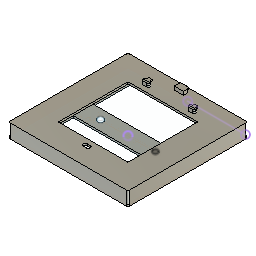
PanaThermoMount (Autodesk Fusion 360 design; units mm, degrees)
part number: 2025-10-30-14-12-04-186
Autodesk Fusion 360 part; units mm, degrees
sketch "MainBoardMount" plane through (0, 0, 0) normal (0, 0, 1) x (1, 0, 0)
  line L0 (0, 60) -> (-58, 60)
  line L1 (-60, 58) -> (-60, -58)
  line L2 (-58, -60) -> (0, -60)
  line L3 (0, 55.6) -> (0, 60)
  line L4 (0, -60) -> (0, -43.8)
  line L5 (0, -39.1) -> (0, 50.6)
  line L6 (0, 60) -> (58, 60)
  line L7 (60, 58) -> (60, -58)
  line L8 (0, -39.1) -> (0, 50.6)
  line L9 (58, -60) -> (0, -60)
  line L10 (0, 55.6) -> (0, 60)
  line L11 (0, -60) -> (0, -43.8)
  arc A0 (60, 58) -> (58, 60) centre (58, 58) ccw
  arc A1 (-58, 60) -> (-60, 58) centre (-58, 58) ccw
  arc A2 (-60, -58) -> (-58, -60) centre (-58, -58) ccw
  arc A3 (58, -60) -> (60, -58) centre (58, -58) ccw
  arc A4 (-24.65, 43.6) -> (-26.6, 41.65) centre (-24.65, 41.65) ccw
  arc A5 (-26.6, 41.65) -> (-24.65, 39.7) centre (-24.65, 41.65) ccw
  line L12 (-24.65, 39.7) -> (-21.35, 39.7)
  arc A6 (-21.35, 39.7) -> (-19.4, 41.65) centre (-21.35, 41.65) ccw
  arc A7 (-19.4, 41.65) -> (-21.35, 43.6) centre (-21.35, 41.65) ccw
  line L13 (-21.35, 43.6) -> (-24.65, 43.6)
  line L14 (21.35, 43.6) -> (24.65, 43.6)
  arc A8 (26.6, 41.65) -> (24.65, 43.6) centre (24.65, 41.65) ccw
  arc A9 (24.65, 39.7) -> (26.6, 41.65) centre (24.65, 41.65) ccw
  line L15 (24.65, 39.7) -> (21.35, 39.7)
  arc A10 (19.4, 41.65) -> (21.35, 39.7) centre (21.35, 41.65) ccw
  arc A11 (21.35, 43.6) -> (19.4, 41.65) centre (21.35, 41.65) ccw
  line L16 (0, 55.2) -> (4.6, 55.2)
  line L17 (4.6, 55.2) -> (4.6, 51)
  line L18 (4.6, 51) -> (0, 51)
  line L19 (-4.6, 51) -> (0, 51)
  line L20 (-4.6, 55.2) -> (-4.6, 51)
  line L21 (0, 55.2) -> (-4.6, 55.2)
  line L22 (0, -39.5) -> (1.65, -39.5)
  arc A12 (3.6, -41.45) -> (1.65, -39.5) centre (1.65, -41.45) ccw
  arc A13 (1.65, -43.4) -> (3.6, -41.45) centre (1.65, -41.45) ccw
  line L23 (1.65, -43.4) -> (0, -43.4)
  line L24 (-1.65, -43.4) -> (0, -43.4)
  arc A14 (-3.6, -41.45) -> (-1.65, -43.4) centre (-1.65, -41.45) ccw
  arc A15 (-1.65, -39.5) -> (-3.6, -41.45) centre (-1.65, -41.45) ccw
  line L25 (0, -39.5) -> (-1.65, -39.5)
  point P0 (-60, -60)
  point P1 (-19, 44)
  point P2 (-27, 44)
  point P3 (-27, 39.3)
  point P4 (-4, -39.1)
  point P5 (-4, -43.8)
  point P6 (27, 44)
  point P7 (4, -43.8)
  point P8 (27, 39.3)
  point P9 (4, -39.1)
  point P10 (19, 44)
  dimension "d21" = 120
  dimension "d24" = 4.7
  dimension "d25" = 8
  dimension "d26" = 60
  dimension "d28" = 4.7
  dimension "d29" = 4
  dimension "d35" = 2
  constraint perpendicular L0 L1
  constraint parallel L0 L2
  constraint parallel L1 L4
  constraint horizontal L0
  constraint coincident L3.start L4
  constraint coincident L5.start L4
  constraint collinear L3 L4
  constraint collinear L4 L5
  constraint symmetric L0.start L5 L3.end
  constraint symmetric L2.end L5 L4.start
  constraint symmetric P1 L5 P10
  constraint symmetric P2 L5 P6
  constraint symmetric P3 L5 P8
  constraint symmetric L3.start L5 L10.start
  constraint symmetric L8.end L5 L5.end
  constraint symmetric L8.start L5 L5.start
  constraint symmetric P4 L5 P9
  constraint symmetric P5 L5 P7
  constraint symmetric L4.end L5 L11.end
  constraint tangent L6 A0
  constraint tangent L7 A0
  constraint tangent L0 A1
  constraint tangent L1 A1
  constraint equal A0 A1
  constraint coincident P0 L1
  constraint coincident P0 L2
  constraint tangent L1 A2
  constraint tangent L2 A2
  constraint equal A0 A2
  constraint tangent L7 A3
  constraint tangent L9 A3
  constraint equal A0 A3
  constraint tangent L22 A12
  constraint tangent L24 A14
  constraint tangent A12 A13
  constraint tangent A13 L23
  constraint tangent A14 A15
  constraint tangent A15 L25
  constraint tangent A4 L13
  constraint tangent A4 A5
  constraint tangent A5 L12
  constraint tangent A6 A7
  constraint tangent L12 A6
  constraint tangent A7 L13
  constraint tangent L14 A11
  constraint tangent L14 A8
  constraint tangent L15 A10
  constraint tangent A8 A9
  constraint tangent A9 L15
  constraint tangent A10 A11
  measures "d21" distance of L0.start L2.end
  measures "d24" distance of P2 P3
  measures "d25" distance of P1 P2
  measures "d26" distance of P0 L2.end
  measures "d28" distance of P4 P5
  measures "d29" distance of L5.start P4
  measures "d35" radius of A0
extrude "Extrude5" add sketch "MainBoardMount" along normal blind 2
sketch "MountingPoints" plane through (0, 0, 2) normal (0, 0, 1) x (-1, 0, 0)
  arc A0 (-24.65, -39.7) -> (-24.65, -43.6) centre (-24.65, -41.65) ccw
  line L0 (-24.65, -39.7) -> (-21.35, -39.7)
  arc A1 (-21.35, -43.6) -> (-21.35, -39.7) centre (-21.35, -41.65) ccw
  line L1 (-21.35, -43.6) -> (-24.65, -43.6)
  line L2 (24.65, -43.6) -> (21.35, -43.6)
  arc A2 (21.35, -39.7) -> (21.35, -43.6) centre (21.35, -41.65) ccw
  line L3 (21.35, -39.7) -> (24.65, -39.7)
  arc A3 (24.65, -43.6) -> (24.65, -39.7) centre (24.65, -41.65) ccw
  arc A4 (-1.65, 43.4) -> (-1.65, 39.5) centre (-1.65, 41.45) ccw
  line L4 (-1.65, 43.4) -> (1.65, 43.4)
  arc A5 (1.65, 39.5) -> (1.65, 43.4) centre (1.65, 41.45) ccw
  line L5 (1.65, 39.5) -> (-1.65, 39.5)
  line L6 (4.6, -55.2) -> (-4.6, -55.2)
  line L7 (-4.6, -55.2) -> (-4.6, -51)
  line L8 (-4.6, -51) -> (4.6, -51)
  line L9 (4.6, -51) -> (4.6, -55.2)
  line L10 (-58, -60) -> (58, -60)
  arc A6 (58, -60) -> (60, -58) centre (58, -58) ccw
  line L11 (60, -58) -> (60, 58)
  arc A7 (60, 58) -> (58, 60) centre (58, 58) ccw
  line L12 (58, 60) -> (-58, 60)
  arc A8 (-58, 60) -> (-60, 58) centre (-58, 58) ccw
  line L13 (-60, 58) -> (-60, -58)
  arc A9 (-60, -58) -> (-58, -60) centre (-58, -58) ccw
extrude "Extrude6" add sketch "MountingPoints" along normal blind 3.5 and the other way blind 2 contours A0 L0 A1 L1 | L2 A2 L3 A3 | L6 L7 L8 L9
sketch "TopmostMountHolder" plane through (0, 55.2, 0) normal (0, 1, 0) x (-1, 0, 0)
  line L0 (-4.6, 2) -> (4.6, 2)
  line L1 (4.6, 2) -> (4.6, 5.5)
  line L2 (4.6, 5.5) -> (-4.6, 5.5)
  line L3 (-4.6, 5.5) -> (-4.6, 2)
  line L4 (-4.6, 5.5) -> (4.6, 5.5)
  line L5 (4.6, 5.5) -> (4.6, 3.75)
  line L6 (4.6, 3.75) -> (-4.6, 3.75)
  line L7 (-4.6, 3.75) -> (-4.6, 5.5)
  dimension "d53" = 1.75
  constraint horizontal L4
  constraint vertical L5
  constraint horizontal L6
  constraint vertical L7
  constraint midpoint L1 L5.end
  constraint coincident L2.end L3.start
  measures "d53" distance of L2.end L6.end
extrude "Extrude7" add sketch "TopmostMountHolder" along normal blind 2 contours L1 L2 L3 L4 L5 L6 L7
fillet "Fillet1" radius 1 1 edges at (0, 57.2, 3.75)
fillet "Fillet2" radius 1 6 edges at (-4.6, 55.7, 3.75) (-4.6, 56.9071, 4.0429) (-4.6, 57.2, 5.125) (4.6, 57.2, 5.125) (4.6, 56.9071, 4.0429) (4.6, 55.7, 3.75)
sketch "FilletedMountHolders" plane through (0, 43.6, 0) normal (0, 1, 0) x (-1, 0, 0)
  line L0 (-24.65, 2) -> (-21.35, 2)
  line L1 (-21.35, 2) -> (-21.35, 5.5)
  line L2 (-21.35, 5.5) -> (-24.65, 5.5)
  line L3 (-24.65, 5.5) -> (-24.65, 2)
ref_plane "WorkPlane1" through (-23, 41.65, 3.75) normal (0, 0, 1) x (-1, 0, 0)
split_face "SplitFace1" 2 faces at (-24.7472, 43.5976, 3.1667) (-19.6147, 40.7604, 3.1667) by plane through (-23, 41.65, 3.75) normal (0, 0, 1)
split_face "SplitFace2" 3 faces at (21.2528, 43.5976, 3.1667) (25.4074, 43.4469, 3.1667) (-22.45, 43.6, 2.5833) by plane through (-23, 41.65, 3.75) normal (0, 0, 1)
split_face "SplitFace3" 1 faces at (22.45, 43.6, 4.3333) by plane through (-23, 41.65, 3.75) normal (0, 0, 1)
ref_plane "WorkPlane2" through (23, 41.65, 3.75) normal (0, -1, 0) x (1, 0, 0)
split_face "SplitFace4" 3 faces at (22.45, 42.3, 5.5) (20.4174, 43.3625, 4.3333) (24.8442, 39.7097, 4.3333) by plane through (23, 41.65, 3.75) normal (0, -1, 0)
split_face "SplitFace5" 2 faces at (22.45, 43.6, 4.3333) (22.45, 43.6, 2.5833) by plane through (-23, 41.65, 3.75) normal (0, 0, 1)
split_face "SplitFace6" 3 faces at (-20.1726, 40.0956, 4.3333) (-23.55, 42.3, 5.5) (-26.0459, 43.0116, 4.3333) by plane through (23, 41.65, 3.75) normal (0, -1, 0)
move_face "OffsetFaces1" offset 2 1 faces at (22.45, 43.6, 4.3333)
move_face "OffsetFaces2" offset 2 1 faces at (-23.55, 43.6, 4.3333)
fillet "Fillet3" radius 1 2 edges at (-23, 45.6, 3.75) (23, 45.6, 3.75)
sketch "BackHole" plane through (0, 0, 0) normal (0, 0, -1) x (1, 0, 0)
  arc A0 (1.65, 39.5) -> (1.65, 43.4) centre (1.65, 41.45) ccw
  line L0 (1.65, 39.5) -> (-1.65, 39.5)
  arc A1 (-1.65, 43.4) -> (-1.65, 39.5) centre (-1.65, 41.45) ccw
  line L1 (-1.65, 43.4) -> (1.65, 43.4)
  line L2 (-58, -60) -> (58, -60)
  arc A2 (58, -60) -> (60, -58) centre (58, -58) ccw
  line L3 (60, -58) -> (60, 58)
  arc A3 (60, 58) -> (58, 60) centre (58, 58) ccw
  line L4 (58, 60) -> (-58, 60)
  arc A4 (-58, 60) -> (-60, 58) centre (-58, 58) ccw
  line L5 (-60, 58) -> (-60, -58)
  arc A5 (-60, -58) -> (-58, -60) centre (-58, -58) ccw
  line L6 (35, -35) -> (-35, -35)
  line L7 (-35, -35) -> (-35, 35)
  line L8 (-35, 35) -> (35, 35)
  line L9 (35, 35) -> (35, -35)
  constraint horizontal L6
  constraint vertical L7
  constraint horizontal L8
  constraint vertical L9
extrude "Extrude8" cut sketch "BackHole" against normal blind 2 contours L6 L7 L8 L9
sketch "Wall" plane through (0, 0, 0) normal (0, 0, -1) x (1, 0, 0)
  line L0 (-35, -35) -> (-35, 35)
  line L1 (-35, 35) -> (35, 35)
  line L2 (35, 35) -> (35, -35)
  line L3 (35, -35) -> (-35, -35)
  arc A0 (1.65, 39.5) -> (1.65, 43.4) centre (1.65, 41.45) ccw
  line L4 (1.65, 39.5) -> (-1.65, 39.5)
  arc A1 (-1.65, 43.4) -> (-1.65, 39.5) centre (-1.65, 41.45) ccw
  line L5 (-1.65, 43.4) -> (1.65, 43.4)
  line L6 (-58, -60) -> (58, -60)
  arc A2 (58, -60) -> (60, -58) centre (58, -58) ccw
  line L7 (60, -58) -> (60, 58)
  arc A3 (60, 58) -> (58, 60) centre (58, 58) ccw
  line L8 (58, 60) -> (-58, 60)
  arc A4 (-58, 60) -> (-60, 58) centre (-58, 58) ccw
  line L9 (-60, 58) -> (-60, -58)
  arc A5 (-60, -58) -> (-58, -60) centre (-58, -58) ccw
  line L10 (58, -58) -> (-58, -58)
  line L11 (-58, -58) -> (-58, 58)
  line L12 (-58, 58) -> (58, 58)
  line L13 (58, 58) -> (58, -58)
  dimension "d63" = 2
  dimension "d64" = 2
  constraint horizontal L10
  constraint vertical L11
  constraint horizontal L12
  constraint vertical L13
  constraint coincident A4.centre L11.end
  constraint coincident A2.centre L10.start
  measures "d63" distance of L6 L10
  measures "d64" distance of L7 L13
extrude "Extrude9" add sketch "Wall" along normal blind 10 contours L6 A2 L7 A3 L8 A4 L9 A5
sketch "BottomPlane" plane through (0, 0, -10) normal (0, 0, -1) x (1, 0, 0)
  line L0 (-58, 58) -> (58, 58)
  line L1 (58, 58) -> (58, -58)
  line L2 (58, -58) -> (-58, -58)
  line L3 (-58, -58) -> (-58, 58)
  arc A0 (-60, -58) -> (-58, -60) centre (-58, -58) ccw
  line L4 (-58, -60) -> (58, -60)
  arc A1 (58, -60) -> (60, -58) centre (58, -58) ccw
  line L5 (60, -58) -> (60, 58)
  arc A2 (60, 58) -> (58, 60) centre (58, 58) ccw
  line L6 (58, 60) -> (-58, 60)
  arc A3 (-58, 60) -> (-60, 58) centre (-58, 58) ccw
  line L7 (-60, 58) -> (-60, -58)
  line L8 (58, -60) -> (-58, -60)
  line L9 (-60, -58) -> (-60, 58)
  line L10 (-58, 60) -> (58, 60)
  line L11 (60, 58) -> (60, -58)
  arc A4 (-60, -58) -> (-58, -60) centre (-58, -58) ccw
  arc A5 (58, -60) -> (60, -58) centre (58, -58) ccw
  arc A6 (60, 58) -> (58, 60) centre (58, 58) ccw
  arc A7 (-58, 60) -> (-60, 58) centre (-58, 58) ccw
  point P0 (60, -60)
  point P1 (-60, -60)
  point P2 (60, 60)
  dimension "d67" = 120
  dimension "d68" = 120
  dimension "d69" = 2
  constraint horizontal L8
  constraint vertical L9
  constraint horizontal L10
  constraint vertical L11
  constraint coincident P1 L8
  constraint coincident P1 L9
  constraint tangent L8 A4
  constraint tangent L9 A4
  constraint coincident P0 L8
  constraint coincident P0 L11
  constraint tangent L8 A5
  constraint tangent L11 A5
  constraint equal A4 A5
  constraint coincident P2 L10
  constraint coincident P2 L11
  constraint tangent L10 A6
  constraint tangent L11 A6
  constraint equal A4 A6
  constraint tangent L9 A7
  constraint tangent L10 A7
  constraint equal A4 A7
  measures "d67" distance of P0 P1
  measures "d68" distance of P0 P2
  measures "d69" radius of A4
extrude "Extrude10" add sketch "BottomPlane" along normal blind 2 contours L0 L1 L2 L3 | A0 L4 A1 L5 A2 L6 A3 L7 L8 L9 L10 L11 A4 A5 A6 A7
sketch "MountingHoles" plane through (0, 0, -10) normal (0, 0, 1) x (-1, 0, 0)
  line L0 (58, -58) -> (58, 58)
  line L1 (58, 58) -> (-58, 58)
  line L2 (-58, 58) -> (-58, -58)
  line L3 (-58, -58) -> (58, -58)
  circle A0 centre (27.5, 0) radius 2.5
  circle A1 centre (-27.5, 0) radius 2.5
  line L4 (0, -60) -> (-58, -60)
  dimension "d91" = 5
  dimension "d92" = 5
  dimension "d93" = 55
  dimension "d94" = 27.5
  dimension "d95" = 60
  measures "d91" diameter of A0
  measures "d92" diameter of A1
  measures "d93" distance of A0.centre A1.centre
  measures "d94" distance of A1.centre origin
  measures "d95" distance of A1.centre L4
hole "Hole3" at (-27.5, 0, -10) direction (0, 0, -1) diameter 3.4 depth 2 tip angle 180 countersink diameter 6.3 countersink angle 90
hole "Hole4" at (27.5, 0, -10) direction (0, 0, -1) diameter 3.4 depth 2 tip angle 180 countersink diameter 6.3 countersink angle 90
sketch "CableBackHole" plane through (0, 0, -12) normal (0, 0, -1) x (1, 0, 0)
  circle A0 centre (27.5, 0) radius 1.7
  circle A1 centre (-27.5, 0) radius 1.7
  arc A2 (60, 58) -> (58, 60) centre (58, 58) ccw
  line L0 (58, 60) -> (-58, 60)
  arc A3 (-58, 60) -> (-60, 58) centre (-58, 58) ccw
  line L1 (-60, 58) -> (-60, -58)
  arc A4 (-60, -58) -> (-58, -60) centre (-58, -58) ccw
  line L2 (-58, -60) -> (58, -60)
  arc A5 (58, -60) -> (60, -58) centre (58, -58) ccw
  line L3 (60, -58) -> (60, 58)
  line L4 (45, 10) -> (-45, 10)
  line L5 (-45, 10) -> (-45, 50)
  line L6 (-45, 50) -> (45, 50)
  line L7 (45, 50) -> (45, 10)
  line L8 (45, -10) -> (-45, -10)
  line L9 (-45, -10) -> (-45, -50)
  line L10 (-45, -50) -> (45, -50)
  line L11 (45, -50) -> (45, -10)
  constraint horizontal L4
  constraint vertical L5
  constraint horizontal L6
  constraint vertical L7
  constraint horizontal L8
  constraint vertical L9
  constraint horizontal L10
  constraint vertical L11
extrude "Extrude11" cut sketch "CableBackHole" against normal blind 2 contours L4 L5 L6 L7 | L8 L9 L10 L11
equation "d94 = ( 55 / 2 ) * 1 mm"
